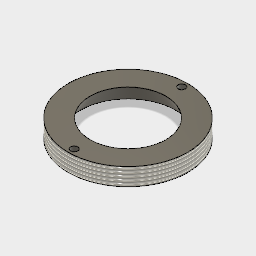
SMB plug dielectric CAM v17 (Autodesk Fusion 360 archive; units mm, degrees)
design "Collet Top Taper"
Autodesk Fusion 360 part; units mm, degrees
sketch "Sketch1" plane through (0, 0, 0) normal (0, 0, 1) x (1, 0, 0)
  line L0 (-20.7744, 0) -> (-26.35, 0)
  line L1 (-26.35, 0) -> (-26.35, 7.62)
  line L2 (-26.35, 7.62) -> (-16.375, 7.62)
  line L3 (-16.375, 7.62) -> (-20.7744, 0)
  dimension "d1" = 26.35
  dimension "d2" = 16.375
  dimension "d3" = 60
  dimension "d4" = 7.62
  dimension "d5" = 7.62
  measures "d1" distance of origin L0.end
  measures "d2" distance of origin L2.end
  measures "d3" angle of L0 L3
  measures "d4" distance of L0.end L1.end
  measures "d5" distance of origin L2.end
sketch "Sketch2" plane through (0, 0, 0) normal (0, 0, 1) x (1, 0, 0)
  line L0 (0, 0) -> (0, 1)
  line L1 (0, 1) -> (0, 14) construction
revolve "Revolve1" add sketch "Sketch1" angle 360 about axis through (0, 1, 0) along (0, 1, 0)
thread "Thread1" "ISO Metric profile 52.0 M52x1.5 6g" major diameter 51.85 minor diameter 50.1269 pitch 1.5 angle 60 resizes the face on face at (-26.2191, 2.54, -2.6236)
sketch "Sketch3" plane through (0, 7.62, 0) normal (0, 1, 0) x (-1, 0, 0)
  circle A0 centre (0, 0) radius 25.925
  circle A1 centre (0, 0) radius 16.375
  point P0 (-0.0141, -23.35)
  point P1 (-0.0141, 23.35)
  dimension "d7" = 46.7
  dimension "d8" = 23.35
  measures "d7" distance of P0 P1
  measures "d8" distance of A0.centre P0
hole "Hole1" at (0.0141, 7.62, -23.35) at (0.0141, 7.62, 23.35) direction (0, -1, 0) diameter 3.1 depth 13.5 tip angle 118
equation "d1 = ( 52.7 / 2 ) * 1 mm"
equation "d2 = ( 32.75 / 2 ) * 1 mm"

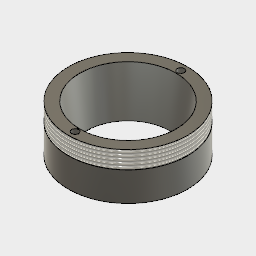
design "Collet Bottom Taper"
Autodesk Fusion 360 part; units mm, degrees
sketch "Sketch1" plane through (0, 0, 0) normal (0, 0, 1) x (1, 0, 0)
  line L0 (-18.15, 0) -> (-25.95, 0)
  line L1 (-25.95, 0) -> (-25.95, 12.7)
  line L2 (-25.95, 12.7) -> (-26.375, 12.7)
  line L3 (-26.375, 12.7) -> (-26.375, 20.32)
  line L4 (-26.375, 20.32) -> (-21.0058, 20.32)
  line L5 (-21.0058, 20.32) -> (-18.15, 0)
  dimension "d1" = 25.95
  dimension "d2" = 26.375
  dimension "d3" = 12.7
  dimension "d4" = 7.62
  dimension "d5" = 98
  dimension "d6" = 7.8
  dimension "d7" = 20.32
  measures "d1" distance of origin L1
  measures "d2" distance of origin L3
  measures "d3" distance of L0.end L1.end
  measures "d4" distance of L2.end L3.end
  measures "d5" angle of L0 L5
  measures "d6" distance of L0.end L0.start
  measures "d7" distance of origin L4.end
sketch "Sketch2" plane through (0, 0, 0) normal (0, 0, 1) x (1, 0, 0)
  line L0 (-18.15, 0) -> (-25.95, 0)
  line L1 (0, 0) -> (0, 22) construction
revolve "Revolve1" add sketch "Sketch1" angle 360 about axis through (0, 0, 0) along (0, 1, 0)
thread "Thread1" "ISO Metric profile 52.0 M52x1.5 6g" major diameter 51.85 minor diameter 50.1269 pitch 1.5 angle 60 resizes the face on face at (-26.3422, 15.24, -1.3147)
sketch "Sketch3" plane through (0, 20.32, 0) normal (0, 1, 0) x (-1, 0, 0)
  circle A0 centre (0, 0) radius 25.925
  circle A1 centre (0, 0) radius 21.0058
  point P0 (0, -23)
  point P1 (0, 23)
  dimension "d9" = 46
  dimension "d10" = 23
  measures "d9" distance of P0 P1
  measures "d10" distance of A0.centre P0
hole "Hole1" at (0, 20.32, -23) at (0, 20.32, 23) direction (0, -1, 0) diameter 3.1 depth 13.5 tip angle 118
equation "d1 = ( 51.9 / 2 ) * 1 mm"
equation "d2 = ( 52.75 / 2 ) * 1 mm"

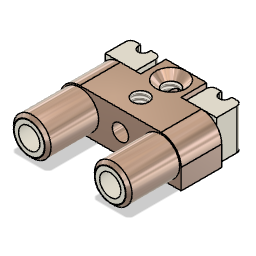
design "SMB plug"
Autodesk Fusion 360 part; units mm, degrees
sketch "Sketch1" plane through (0, 0, 0) normal (0, 0, 1) x (1, 0, 0)
  circle A0 centre (-4, 0) radius 1.85
  circle A1 centre (4, 0) radius 1.85
  line L0 (0, 1.75) -> (0, 22.5) construction
  line L1 (1.75, 0) -> (22.5, 0) construction
  line L2 (-6, -2) -> (6, -2)
  line L3 (6, -2) -> (6, 2)
  line L4 (6, 2) -> (-6, 2)
  line L5 (-6, 2) -> (-6, -2)
  circle A2 centre (-4, 0) radius 1.5
  circle A3 centre (4, 0) radius 1.55
  line L6 (-2, 2) -> (-2, -2)
  line L7 (2, 2) -> (2, -2)
  circle A4 centre (-4, 0) radius 1.05
  circle A5 centre (-4, 0) radius 0.25
  dimension "d2" = 3.7
  dimension "d3" = 3.7
  dimension "d4" = 8
  dimension "d5" = 12
  dimension "d6" = 2
  dimension "d7" = 4
  dimension "d12" = -0.35
  dimension "d13" = -0.3
  dimension "d26" = 4
  dimension "d37" = 2.1
  dimension "d38" = 0.5
  constraint symmetric A0.centre A1.centre L0
  constraint coincident A1.centre L1
  constraint horizontal L2
  constraint perpendicular L1 L3
  constraint perpendicular L3 L4
  constraint perpendicular L2 L5
  constraint symmetric L0 L3 L5
  constraint coincident L4 L6.start
  constraint coincident L2 L6.end
  constraint perpendicular L2 L6
  constraint coincident L4 L7.start
  constraint coincident L2 L7.end
  constraint perpendicular L2 L7
  constraint symmetric L0 L6 L7
  constraint concentric A0 A4
  constraint concentric A4 A5
  measures "d2" diameter of A0
  measures "d3" diameter of A1
  measures "d4" distance of A0.centre A1.centre
  measures "d5" distance of L3 L5
  measures "d6" distance of L1 L2
  measures "d7" distance of L2 L4
  measures "d26" distance of L6 L7
  measures "d37" diameter of A4
  measures "d38" diameter of A5
extrude "Extrude1" add sketch "Sketch1" along normal blind 5 contours A0 | A1 | A2 | A3 | A4 | A5 makes body 1 at (-2.1523, -0.0922, 3.3333) makes body 2 at (5.8477, -0.0922, 3.3333)
extrude "Extrude2" add sketch "Sketch1" against normal blind 4 contours A0 | A1 | L2 L4 L5 L6 | L2 L4 L6 L7 | L2 L3 L4 L7 | A2 | A3 | A4 | A5 bodies 1 2
extrude "Extrude3" cut sketch "Sketch1" along normal through all and the other way through all contours A2 | A3 | A4 | A5 bodies 1
extrude "Extrude4" add sketch "Sketch1" against normal blind 6.5 contours L2 L4 L6 L7 bodies 1
chamfer "Chamfer1" distance 0.3 angle 45 2 edges at (-5.7248, -0.669, 5) (2.2752, -0.669, 5) on bodies 1
sketch "Sketch2" plane through (0, 2, 0) normal (0, 1, 0) x (-1, 0, 0)
  line L0 (6, 0) -> (-6, 0)
  line L1 (-6, 0) -> (-6, -4)
  line L2 (2, -4) -> (6, -4)
  line L3 (6, -4) -> (6, 0)
  line L4 (0, 0) -> (0, -6.5) construction
  line L5 (-6, -4) -> (-2, -4)
  line L6 (-2, -4) -> (-2, -6.5)
  line L7 (-2, -6.5) -> (2, -6.5)
  line L8 (2, -6.5) -> (2, -4)
  line L9 (-6, 0) -> (6, 0)
  point P0 (0, -2)
  point P1 (0, -5)
  dimension "d29" = 2
  dimension "d36" = 5
  constraint coincident L4.start origin
  constraint midpoint L4.end L7
  constraint coincident L4 P1
  measures "d29" distance of L4.start P0
  measures "d36" distance of P1 L9
extrude "Extrude5" add sketch "Sketch1" along normal up to surface (-4 mm away) and the other way up to surface (-5 mm away) separate body contours A2 | A4 makes body 3
extrude "Extrude6" cut sketch "Sketch1" against normal blind 3.4 from surface at 5 contours A4 bodies 3
hole "Hole1" at (0, 2, -2) direction (0, -1, 0) diameter 1.623 end through all bodies 1
thread "Thread1" "ISO Metric profile 2.0 M2x0.4 6H"
fillet "Fillet1" radius 2 2 edges at (6, 2, -2) (-6, 2, -2) on bodies 1
hole "Hole2" at (0, 0, 0) direction (0, 0, -1) diameter 1.6 depth 9 tip angle 118 bodies 1
hole "Hole3" at (0, 2, -5) direction (0, -1, 0) diameter 1.623 depth 5 tip angle 118 countersink diameter 3 countersink angle 90 bodies 1
thread "Thread2" "ISO Metric profile 2.0 M2x0.4 6H"
sketch "Sketch3" plane through (0, 0, -4) normal (0, 0, -1) x (-1, 0, 0)
  circle A0 centre (4, 0) radius 0.25
  circle A1 centre (4, 0) radius 1.5
  line L0 (2.5, 2) -> (5.5, 2)
  line L1 (5.5, 2) -> (5.5, -2)
  line L2 (5.5, -2) -> (2.5, -2)
  line L3 (2.5, -2) -> (2.5, 2)
  circle A2 centre (4, 0) radius 1.5
  constraint horizontal L0
  constraint vertical L1
  constraint horizontal L2
  constraint vertical L3
  constraint tangent L3 A2
  constraint tangent L1 A2
extrude "Extrude7" add sketch "Sketch3" along normal blind 2.5 bodies 3
fillet "Fillet3" [suppressed]
sketch "Sketch6" plane through (0, 2, 0) normal (0, 1, 0) x (-1, 0, 0)
  line L0 (5.5, -6.5) -> (5.5, -4)
  line L1 (5.5, -4) -> (2.5, -4)
  line L2 (2.5, -4) -> (2.5, -6.5)
  line L3 (2.5, -6.5) -> (5.5, -6.5)
  line L4 (4, 0) -> (4, -6.9)
  line L5 (3.5, -6.5) -> (3.5, -6.25)
  arc A0 (4.5, -6.25) -> (3.5, -6.25) centre (4, -6.25) ccw
  line L6 (4.5, -6.25) -> (4.5, -6.5)
  point P0 (4, 0)
  dimension "d49" = 1
  dimension "d50" = 0.25
  constraint coincident P0 L4.start
  constraint perpendicular L3 L4
  constraint coincident L3 L5.start
  constraint perpendicular L3 L5
  constraint tangent L5 A0
  constraint tangent A0 L6
  constraint parallel L4 L6
  constraint coincident L4 A0.centre
  constraint coincident L3 L6.end
  measures "d49" distance of L5 L6
  measures "d50" distance of L3 A0.centre
extrude "Extrude8" cut sketch "Sketch6" against normal blind 2.5 contours L3 L4 A0 L6 | L3 L4 L5 A0 bodies 3
fillet "Fillet4" radius 0.5 2 edges at (-2.5, 0, -6.5) (-5.5, 0, -6.5) on bodies 3
mirror "Mirror1" about plane through (0, 0, 0) normal (1, 0, 0) of bodies 3 makes body 4
copy_body "Body->Comp1" bodies 1 removing the originals makes body 5 in component "connector"
copy_body "Body->Comp2" bodies 3 removing the originals makes body 6 in component "R dielectric"
copy_body "Body->Comp3" bodies 4 removing the originals makes body 7 in component "L dielectric"
component "connector" placed x (1, 0, 0) y (0, 1, 0) z (0, 0, 1) at (0, 0, 0)
component "R dielectric" placed x (1, 0, 0) y (0, 1, 0) z (0, 0, 1) at (0, 0, 0)
component "L dielectric" placed x (1, 0, 0) y (0, 1, 0) z (0, 0, 1) at (0, 0, 0)
named bodies: "connector", "R dielectric", "L dielectric"
